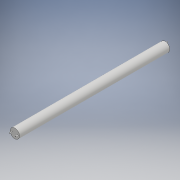
# Autodesk Inventor part: UV-15W
Saved by Autodesk Inventor 2017 (Build 210142000, 142)
## iProperties
Created: 2021-01-04
Part Number: UV-15W
Material: Generic
Document SubType Name: Modeling
Designer: USUARIO
Density: 1 g/cm^3
Appearance: Default
Author: USUARIO
Autodesk Inventor part; units mm, degrees
ref_plane "YZ Plane" through (0, 0, 0) normal (1, 0, 0) x (0, 1, 0)
ref_plane "XZ Plane" through (0, 0, 0) normal (0, 1, 0) x (-1, 0, 0)
ref_plane "XY Plane" through (0, 0, 0) normal (0, 0, 1) x (1, 0, 0)
sketch "Sketch1" plane through (0, 0, 0) normal (0, 1, 0) x (-1, 0, 0)
  circle A0 centre (0, 0) radius 13.5
  dimension "d0" = 27
  constraints: 1 centre point, 1 coincident
  measures "d0" diameter of A0
extrude "Extrusion1" add sketch "Sketch1" along normal blind 436
sketch "Sketch2" plane through (0, 436, 0) normal (0, 1, 0) x (1, 0, 0)
  circle A0 centre (0, -8.8) radius 1
  circle A1 centre (0, 8.8) radius 1
  circle A2 centre (0, 0) radius 13.5 projected
  dimension "d3" = 2
  dimension "d4" = 2
  dimension "d5" = 8.8
  dimension "d6" = 8.8
  constraints: 2 centre point
  measures "d3" diameter of A0
  measures "d4" diameter of A1
  measures "d5" distance of A2.centre A1.centre
  measures "d6" distance of A2.centre A0.centre
extrude "Extrusion2" add sketch "Sketch2" along normal blind 7 contours A0 | A1
sketch "Sketch3" plane through (0, 0, 0) normal (0, -1, 0) x (1, 0, 0)
  circle A0 centre (-8.8, 0) radius 1
  circle A1 centre (8.8, 0) radius 1
  point P0 (0, 0)
  dimension "d9" = 2
  dimension "d10" = 2
  dimension "d11" = 8.8
  dimension "d12" = 8.8
  constraints: 2 centre point
  measures "d9" diameter of A0
  measures "d10" diameter of A1
  measures "d11" distance of point (0, 0) A0.centre
  measures "d12" distance of point (0, 0) A1.centre
extrude "Extrusion3" add sketch "Sketch3" along normal blind 7
body "Solid1"
